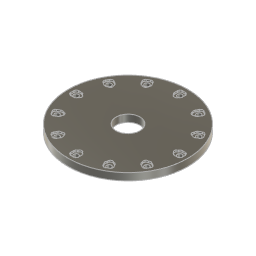
disk v1 (Autodesk Fusion 360 design; units mm, degrees)
Autodesk Fusion 360 part; units mm, degrees
sketch "Sketch1" plane through (0, 0, 0) normal (0, 0, 1) x (1, 0, 0)
  circle A0 centre (0, 0) radius 75
  dimension "d1" = 150
  constraint coincident A0.centre origin
  measures "d1" diameter of A0
extrude "Extrude1" add sketch "Sketch1" along normal blind 9
sketch "Sketch2" plane through (0, 0, 9) normal (0, 0, 1) x (-1, 0, 0)
  circle A0 centre (0, 0) radius 75
  circle A1 centre (0, 0) radius 15
  circle A2 centre (0, -65) radius 3
  circle A3 centre (32.5, -56.2917) radius 3
  circle A4 centre (56.2917, -32.5) radius 3
  circle A5 centre (65, 0) radius 3
  circle A6 centre (56.2917, 32.5) radius 3
  circle A7 centre (32.5, 56.2917) radius 3
  circle A8 centre (0, 65) radius 3
  circle A9 centre (-32.5, 56.2917) radius 3
  circle A10 centre (-56.2917, 32.5) radius 3
  circle A11 centre (-65, 0) radius 3
  circle A12 centre (-56.2917, -32.5) radius 3
  circle A13 centre (-32.5, -56.2917) radius 3
  circle A14 centre (0, 0) radius 65 construction
  dimension "d4" = 30
  dimension "d10" = 360
  dimension "d14" = 6
  constraint coincident A0.centre A1.centre
  constraint coincident A2.centre A14
  measures "d4" diameter of A1
  measures "d14" diameter of A2
extrude "Extrude2" cut sketch "Sketch2" against normal blind 40 contours A1 | A2 | A3 | A4 | A5 | A6 | A7 | A8 | A9 | A10 | A11 | A12 | A13
sketch "Sketch3" plane through (0, 0, 9) normal (0, 0, 1) x (-1, 0, 0)
  circle A0 centre (0, 0) radius 15
  circle A1 centre (-32.5, 56.2917) radius 3
  circle A2 centre (0, 65) radius 3
  circle A3 centre (0, -65) radius 3
  circle A4 centre (32.5, -56.2917) radius 3
  circle A5 centre (56.2917, -32.5) radius 3
  circle A6 centre (65, 0) radius 3
  circle A7 centre (-56.2917, 32.5) radius 3
  circle A8 centre (32.5, 56.2917) radius 3
  circle A9 centre (56.2917, 32.5) radius 3
  circle A10 centre (-65, 0) radius 3
  circle A11 centre (0, 0) radius 75
  line L0 (5, -63) -> (5, -67.1292)
  line L1 (2, -70.1292) -> (-2, -70.1292)
  line L2 (-5, -67.1292) -> (-5, -63)
  arc A12 (2, -70.1292) -> (5, -67.1292) centre (2, -67.1292) ccw
  arc A13 (-5, -67.1292) -> (-2, -70.1292) centre (-2, -67.1292) ccw
  arc A14 (-2.8708, -60.1292) -> (-5, -63) centre (-2, -63) ccw
  arc A15 (5, -63) -> (2.8708, -60.1292) centre (2, -63) ccw
  arc A16 (2.8708, -60.1292) -> (-2.8708, -60.1292) centre (0, -61) ccw
  line L3 (29.2345, -60.6356) -> (27.1699, -57.0596)
  arc A17 (27.5784, -53.5088) -> (27.1699, -57.0596) centre (29.7679, -55.5596) ccw
  arc A18 (32.5508, -50.638) -> (27.5784, -53.5088) centre (30.5, -52.8275) ccw
  circle A19 centre (32.5, -56.2917) radius 3
  arc A20 (35.8301, -52.0596) -> (32.5508, -50.638) centre (33.2321, -53.5596) ccw
  line L4 (35.8301, -52.0596) -> (37.8947, -55.6356)
  arc A21 (29.2345, -60.6356) -> (33.3325, -61.7336) centre (31.8325, -59.1356) ccw
  line L5 (36.7966, -59.7336) -> (33.3325, -61.7336)
  arc A22 (36.7966, -59.7336) -> (37.8947, -55.6356) centre (35.2966, -57.1356) ccw
  line L6 (55.6356, -37.8947) -> (52.0596, -35.8301)
  arc A23 (50.638, -32.5508) -> (52.0596, -35.8301) centre (53.5596, -33.2321) ccw
  arc A24 (53.5088, -27.5784) -> (50.638, -32.5508) centre (52.8275, -30.5) ccw
  circle A25 centre (56.2917, -32.5) radius 3
  arc A26 (57.0596, -27.1699) -> (53.5088, -27.5784) centre (55.5596, -29.7679) ccw
  line L7 (57.0596, -27.1699) -> (60.6356, -29.2345)
  arc A27 (55.6356, -37.8947) -> (59.7336, -36.7966) centre (57.1356, -35.2966) ccw
  line L8 (61.7336, -33.3325) -> (59.7336, -36.7966)
  arc A28 (61.7336, -33.3325) -> (60.6356, -29.2345) centre (59.1356, -31.8325) ccw
  line L9 (67.1292, -5) -> (63, -5)
  arc A29 (60.1292, -2.8708) -> (63, -5) centre (63, -2) ccw
  arc A30 (60.1292, 2.8708) -> (60.1292, -2.8708) centre (61, 0) ccw
  circle A31 centre (65, 0) radius 3
  arc A32 (63, 5) -> (60.1292, 2.8708) centre (63, 2) ccw
  line L10 (63, 5) -> (67.1292, 5)
  arc A33 (67.1292, -5) -> (70.1292, -2) centre (67.1292, -2) ccw
  line L11 (70.1292, 2) -> (70.1292, -2)
  arc A34 (70.1292, 2) -> (67.1292, 5) centre (67.1292, 2) ccw
  line L12 (60.6356, 29.2345) -> (57.0596, 27.1699)
  arc A35 (53.5088, 27.5784) -> (57.0596, 27.1699) centre (55.5596, 29.7679) ccw
  arc A36 (50.638, 32.5508) -> (53.5088, 27.5784) centre (52.8275, 30.5) ccw
  circle A37 centre (56.2917, 32.5) radius 3
  arc A38 (52.0596, 35.8301) -> (50.638, 32.5508) centre (53.5596, 33.2321) ccw
  line L13 (52.0596, 35.8301) -> (55.6356, 37.8947)
  arc A39 (60.6356, 29.2345) -> (61.7336, 33.3325) centre (59.1356, 31.8325) ccw
  line L14 (59.7336, 36.7966) -> (61.7336, 33.3325)
  arc A40 (59.7336, 36.7966) -> (55.6356, 37.8947) centre (57.1356, 35.2966) ccw
  line L15 (37.8947, 55.6356) -> (35.8301, 52.0596)
  arc A41 (32.5508, 50.638) -> (35.8301, 52.0596) centre (33.2321, 53.5596) ccw
  arc A42 (27.5784, 53.5088) -> (32.5508, 50.638) centre (30.5, 52.8275) ccw
  circle A43 centre (32.5, 56.2917) radius 3
  arc A44 (27.1699, 57.0596) -> (27.5784, 53.5088) centre (29.7679, 55.5596) ccw
  line L16 (27.1699, 57.0596) -> (29.2345, 60.6356)
  arc A45 (37.8947, 55.6356) -> (36.7966, 59.7336) centre (35.2966, 57.1356) ccw
  line L17 (33.3325, 61.7336) -> (36.7966, 59.7336)
  arc A46 (33.3325, 61.7336) -> (29.2345, 60.6356) centre (31.8325, 59.1356) ccw
  line L18 (5, 67.1292) -> (5, 63)
  arc A47 (2.8708, 60.1292) -> (5, 63) centre (2, 63) ccw
  arc A48 (-2.8708, 60.1292) -> (2.8708, 60.1292) centre (0, 61) ccw
  circle A49 centre (0, 65) radius 3
  arc A50 (-5, 63) -> (-2.8708, 60.1292) centre (-2, 63) ccw
  line L19 (-5, 63) -> (-5, 67.1292)
  arc A51 (5, 67.1292) -> (2, 70.1292) centre (2, 67.1292) ccw
  line L20 (-2, 70.1292) -> (2, 70.1292)
  arc A52 (-2, 70.1292) -> (-5, 67.1292) centre (-2, 67.1292) ccw
  line L21 (-29.2345, 60.6356) -> (-27.1699, 57.0596)
  arc A53 (-27.5784, 53.5088) -> (-27.1699, 57.0596) centre (-29.7679, 55.5596) ccw
  arc A54 (-32.5508, 50.638) -> (-27.5784, 53.5088) centre (-30.5, 52.8275) ccw
  circle A55 centre (-32.5, 56.2917) radius 3
  arc A56 (-35.8301, 52.0596) -> (-32.5508, 50.638) centre (-33.2321, 53.5596) ccw
  line L22 (-35.8301, 52.0596) -> (-37.8947, 55.6356)
  arc A57 (-29.2345, 60.6356) -> (-33.3325, 61.7336) centre (-31.8325, 59.1356) ccw
  line L23 (-36.7966, 59.7336) -> (-33.3325, 61.7336)
  arc A58 (-36.7966, 59.7336) -> (-37.8947, 55.6356) centre (-35.2966, 57.1356) ccw
  line L24 (-55.6356, 37.8947) -> (-52.0596, 35.8301)
  arc A59 (-50.638, 32.5508) -> (-52.0596, 35.8301) centre (-53.5596, 33.2321) ccw
  arc A60 (-53.5088, 27.5784) -> (-50.638, 32.5508) centre (-52.8275, 30.5) ccw
  circle A61 centre (-56.2917, 32.5) radius 3
  arc A62 (-57.0596, 27.1699) -> (-53.5088, 27.5784) centre (-55.5596, 29.7679) ccw
  line L25 (-57.0596, 27.1699) -> (-60.6356, 29.2345)
  arc A63 (-55.6356, 37.8947) -> (-59.7336, 36.7966) centre (-57.1356, 35.2966) ccw
  line L26 (-61.7336, 33.3325) -> (-59.7336, 36.7966)
  arc A64 (-61.7336, 33.3325) -> (-60.6356, 29.2345) centre (-59.1356, 31.8325) ccw
  line L27 (-67.1292, 5) -> (-63, 5)
  arc A65 (-60.1292, 2.8708) -> (-63, 5) centre (-63, 2) ccw
  arc A66 (-60.1292, -2.8708) -> (-60.1292, 2.8708) centre (-61, 0) ccw
  circle A67 centre (-65, 0) radius 3
  arc A68 (-63, -5) -> (-60.1292, -2.8708) centre (-63, -2) ccw
  line L28 (-63, -5) -> (-67.1292, -5)
  arc A69 (-67.1292, 5) -> (-70.1292, 2) centre (-67.1292, 2) ccw
  line L29 (-70.1292, -2) -> (-70.1292, 2)
  arc A70 (-70.1292, -2) -> (-67.1292, -5) centre (-67.1292, -2) ccw
  line L30 (-60.6356, -29.2345) -> (-57.0596, -27.1699)
  arc A71 (-53.5088, -27.5784) -> (-57.0596, -27.1699) centre (-55.5596, -29.7679) ccw
  arc A72 (-50.638, -32.5508) -> (-53.5088, -27.5784) centre (-52.8275, -30.5) ccw
  circle A73 centre (-56.2917, -32.5) radius 3
  arc A74 (-52.0596, -35.8301) -> (-50.638, -32.5508) centre (-53.5596, -33.2321) ccw
  line L31 (-52.0596, -35.8301) -> (-55.6356, -37.8947)
  arc A75 (-60.6356, -29.2345) -> (-61.7336, -33.3325) centre (-59.1356, -31.8325) ccw
  line L32 (-59.7336, -36.7966) -> (-61.7336, -33.3325)
  arc A76 (-59.7336, -36.7966) -> (-55.6356, -37.8947) centre (-57.1356, -35.2966) ccw
  line L33 (-37.8947, -55.6356) -> (-35.8301, -52.0596)
  arc A77 (-32.5508, -50.638) -> (-35.8301, -52.0596) centre (-33.2321, -53.5596) ccw
  arc A78 (-27.5784, -53.5088) -> (-32.5508, -50.638) centre (-30.5, -52.8275) ccw
  circle A79 centre (-32.5, -56.2917) radius 3
  arc A80 (-27.1699, -57.0596) -> (-27.5784, -53.5088) centre (-29.7679, -55.5596) ccw
  line L34 (-27.1699, -57.0596) -> (-29.2345, -60.6356)
  arc A81 (-37.8947, -55.6356) -> (-36.7966, -59.7336) centre (-35.2966, -57.1356) ccw
  line L35 (-33.3325, -61.7336) -> (-36.7966, -59.7336)
  arc A82 (-33.3325, -61.7336) -> (-29.2345, -60.6356) centre (-31.8325, -59.1356) ccw
  circle A83 centre (-32.5, -56.2917) radius 3
  circle A84 centre (-56.2917, -32.5) radius 3
  point P0 (0, -65)
  point P1 (32.5, -56.2917)
  point P2 (56.2917, -32.5)
  point P3 (65, 0)
  point P4 (56.2917, 32.5)
  point P5 (32.5, 56.2917)
  point P6 (0, 65)
  point P7 (-32.5, 56.2917)
  point P8 (-56.2917, 32.5)
  point P9 (-65, 0)
  point P10 (-56.2917, -32.5)
  point P11 (-32.5, -56.2917)
  dimension "d18" = 3
  dimension "d19" = 4
  dimension "d20" = 10
  dimension "d21" = 10
  dimension "d22" = 3
  dimension "d24" = 360
  constraint parallel L0 L2
  constraint coincident P0 A3.centre
  constraint tangent L0 A12
  constraint tangent L1 A12
  constraint tangent L1 A13
  constraint tangent L2 A13
  constraint equal A12 A13
  constraint tangent L2 A14
  constraint equal A12 A14
  constraint tangent L0 A15
  constraint equal A12 A15
  measures "d18" radius of A12
  measures "d19" distance of P0 A16.centre
  measures "d20" distance of L0 L2
  measures "d21" distance of L1 A14.start
  measures "d22" radius of A16
extrude "Extrude3" cut sketch "Sketch3" against normal blind 2 contours L0 L1 L2 A12 A13 A14 A15 A16 | L3 A17 A18 A20 L4 A21 L5 A22 | L6 A23 A24 A26 L7 A27 L8 A28 | L9 A29 A30 A32 L10 A33 L11 A34 | L12 A35 A36 A38 L13 A39 L14 A40 | L15 A41 A42 A44 L16 A45 L17 A46 | L18 A47 A48 A50 L19 A51 L20 A52 | L21 A53 A54 A56 L22 A57 L23 A58 | L24 A59 A60 A62 L25 A63 L26 A64 | L27 A65 A66 A68 L28 A69 L29 A70 | L30 A71 A72 A74 L31 A75 L32 A76 | L33 A77 A78 A80 L34 A81 L35 A82
equation "d2 = thickness"
equation "amountofobjects = 12"
equation "d9 = amountofobjects"
equation "thickness = 9 mm"
equation "d14 = tooldiameter"
equation "tooldiameter = 6 mm"
equation "d23 = amountofobjects"
